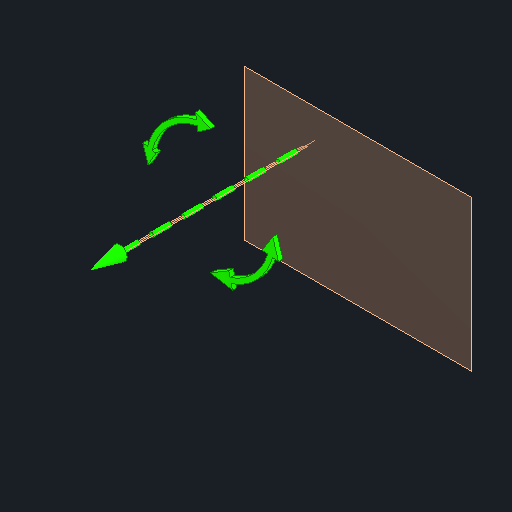
# Autodesk Inventor part: Ось_Схематично
Saved by Autodesk Inventor 2026 (Build 300175000, 175)
## iProperties
Created: 2026-04-19
Part Number: Ось_Схематично
Material: Типовые
Document SubType Name: Modeling
Designer: Artem Sannikov
Density: 1 g/cm^3
Appearance: По умолчанию
Author: Artem Sannikov
Autodesk Inventor part; units mm, degrees
ref_plane "YZ Plane" through (0, 0, 0) normal (1, 0, 0) x (0, 1, 0)
ref_plane "XZ Plane" through (0, 0, 0) normal (0, 1, 0) x (-1, 0, 0)
ref_plane "XY Plane" through (0, 0, 0) normal (0, 0, 1) x (1, 0, 0)
ref_plane "РабПлоскость1" through (0, 0, 0) normal (0, 0, 1) x (1, 0, 0)
sketch "Эскиз1" plane through (0, 0, 0) normal (0, 0, 1) x (1, 0, 0)
  circle A0 centre (-98.3223, 43.4037) radius 9.5 projected
  circle A1 centre (-98.3223, 43.4037) radius 3.5
  point P0 (0, 0)
  dimension "d0" = 7
  constraints: 1 centre point, 1 coincident
  measures "d0" diameter of A1
extrude "Выдавливание1" add sketch "Эскиз1" along normal blind 28.75 contours A1
pattern_linear "Прямоуг.массив1" count 6 spacing 50 along (0, 0, 1) of "Выдавливание1"
ref_plane "РабПлоскость3" through (-98.3223, 43.4037, 250) normal (-0.4330112, 0.9013886, 0) x (0, 0, 1)
ref_plane "РабПлоскость2" through (-312.9172, 686.9729, -45) normal (0.9013886, 0.4330112, 0) x (0.4330112, -0.9013886, 0)
sketch "Эскиз2" plane through (-98.3223, 43.4037, 250) normal (-0.4330112, 0.9013886, 0) x (0, 0, 1)
  line L0 (28.75, -3.5) -> (28.75, 3.5) projected
  line L1 (28.75, 0) -> (28.75, -11.2136)
  line L2 (28.75, -11.2136) -> (77.1017, 0)
  line L3 (77.1017, 0) -> (28.75, 0)
  line L4 (-313.7567, 0) -> (132.5402, 0) projected
  point P0 (-250, 69.8323)
  constraints: 6 end point, 1 midpoint, 1 perpendicular, 1 point on line, 1 vertical
revolve "Вращение1" add sketch "Эскиз2" angle 360 about axis through (-98.3223, 43.4037, 250) along (0, 0, 1)
sketch "Эскиз3" plane through (-98.3223, 43.4037, 128.75) normal (0, 0, 1) x (1, 0, 0)
  circle A0 centre (0, 0) radius 3.5 projected
  circle A1 centre (0, 0) radius 102.5
  circle A2 centre (0, 0) radius 95
  line L0 (0, 102.5) -> (0, 95)
  circle A3 centre (0, 0) radius 11.2136 projected
  line L1 (0, 0) -> (102.5, 0)
  line L2 (0, 0) -> (0, -102.5)
  line L3 (0, -102.5) -> (0, -95)
  line L4 (0, -98.75) -> (29.1539, -81.4588)
  line L5 (29.1539, -81.4588) -> (35.0002, -105.069)
  line L6 (35.0002, -105.069) -> (0, -98.75)
  line L7 (102.5, 0) -> (95, 0)
  line L8 (98.75, 0) -> (107.8547, -29.5163)
  line L9 (107.8547, -29.5163) -> (81.9958, -26.5931)
  line L10 (81.9958, -26.5931) -> (98.75, 0)
  line L11 (-95, 0) -> (-102.5, 0)
  line L12 (0, 102.5) -> (0, 95)
  line L13 (-98.75, 0) -> (-86.2844, 22.2665)
  line L14 (-86.2844, 22.2665) -> (-107.1199, 26.0282)
  line L15 (-107.1199, 26.0282) -> (-98.75, 0)
  line L16 (0, 98.75) -> (-20.0594, 84.1732)
  line L17 (-20.0594, 84.1732) -> (-23.4202, 109.8884)
  line L18 (-23.4202, 109.8884) -> (0, 98.75)
  point P0 (98.3223, -43.4037)
  point P1 (-92.0945, 23.3154)
  point P2 (-21.1624, 92.6129)
  point P3 (-22.1384, 100.0807)
  point P4 (-99.4916, 24.6509)
  point P5 (90.9024, -27.5999)
  point P6 (31.2019, -89.7298)
  point P7 (33.0117, -97.0385)
  point P8 (98.471, -28.4555)
  dimension "d8" = 190
  dimension "d9" = 205
  constraints: 38 end point, 8 point on circle, 4 midpoint, 2 centre point, 2 coincident, 2 horizontal, 2 perpendicular, 2 point on line
  measures "d8" diameter of A2
  measures "d9" diameter of A1
extrude "Выдавливание2" add sketch "Эскиз3" along normal blind 7 contours L10 L8 A1 L9 A2 | A2 L9 L10 | L4 L5 A2 | A2 L5 A1 L6 L4 | L16 L17 A2 | A2 L17 A1 L18 L16 | L9 A1 L5 A2 | L8 L9 A1 | L13 L15 A1 L14 A2 | A2 L14 L13 | A1 L5 L6 | A2 L14 A1 L17 | A1 L17 L18 | L15 L14 A1
